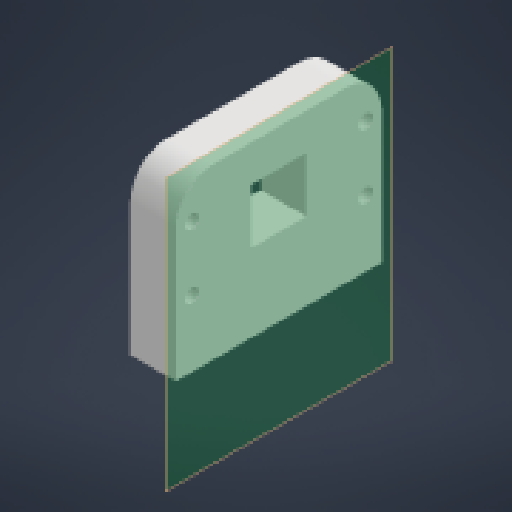
# Autodesk Inventor part: upper_cup
Saved by Autodesk Inventor 2024 (Build 280153000, 153)
## iProperties
Created: 2023-11-08
Part Number: upper_cup
Material: Типовые
Document SubType Name: Modeling
Designer: user
Density: 1 g/cm^3
Appearance: По умолчанию
Author: user
Autodesk Inventor part; units mm, degrees
ref_plane "YZ Plane" through (0, 0, 0) normal (1, 0, 0) x (0, 1, 0)
ref_plane "XZ Plane" through (0, 0, 0) normal (0, 1, 0) x (-1, 0, 0)
ref_plane "XY Plane" through (0, 0, 0) normal (0, 0, 1) x (1, 0, 0)
ref_plane "РабПлоскость1" through (-32.5, 0, 7) normal (-1, 0, 0) x (0, 1, 0)
sketch "Эскиз1" plane through (-32.5, 0, 7) normal (-1, 0, 0) x (0, 1, 0)
  line L0 (15, -5) -> (15, -24) projected
  arc A0 (15, -5) -> (15, 5) centre (15, 0) ccw projected
  line L1 (15, -24) -> (-15, -24) projected
  arc A1 (14.5, -30) -> (22.5, -22) centre (14.5, -22) ccw projected
  line L2 (-14.5, -30) -> (14.5, -30) projected
  arc A2 (-22.5, -22) -> (-14.5, -30) centre (-14.5, -22) ccw projected
  circle A3 centre (-19, -21.5) radius 1.5 projected
  circle A4 centre (-19, -7.5) radius 1.5 projected
  circle A5 centre (19, -21.5) radius 1.5 projected
  circle A6 centre (19, -7.5) radius 1.5 projected
  line L3 (-15, -24) -> (-15, 24) construction
  line L4 (-22.5, 24) -> (-22.5, -22) construction
  line L5 (22.5, -22) -> (22.5, 24) construction
  line L6 (15, 24) -> (15, 5) construction
  line L7 (22.5, -22) -> (22.5, 7)
  line L8 (14, 7) -> (-14, 7) projected
  line L9 (14, 7) -> (22.5, 7)
  line L10 (-14, 7) -> (-15, 7)
  line L11 (-15, 7) -> (-15, -24)
  line L12 (-22.5, -22) -> (-22.5, 7)
  line L13 (-22.5, 7) -> (-15, 7)
  line L14 (15, 5) -> (15, 7)
  line L15 (-6, -22) -> (6, -22)
  line L16 (6, -22) -> (6, -10)
  line L17 (6, -10) -> (-6, -10)
  line L18 (-6, -10) -> (-6, -22)
  point P0 (0, 7)
  point P1 (0, -10)
  dimension "d0" = 2
  dimension "d1" = 12
  dimension "d2" = 12
  constraints: 22 end point, 7 point on line, 3 perpendicular, 2 parallel, 1 collinear, 1 horizontal, 1 midpoint, 1 vertical alignment
  measures "d0" vertical distance of L1.end L15.start
  measures "d1" distance of L16.end L17.end
  measures "d2" distance of L17.end L15.start
extrude "Выдавливание1" add sketch "Эскиз1" along normal blind 10
sketch "Эскиз2" plane through (-32.5, -22.5, 0) normal (0, 0, -1) x (-1, 0, 0)
  arc A0 (7, 34.4641) -> (7, 27.5359) centre (5, 31) ccw projected
  arc A1 (7, 17.4641) -> (7, 10.5359) centre (5, 14) ccw projected
  arc A2 (7, 27.5359) -> (7, 34.4641) centre (5, 31) ccw
  arc A3 (7, 10.5359) -> (7, 17.4641) centre (5, 14) ccw
  point P0 (-32.5, 22.5)
  constraints: 4 point on circle, 2 centre point, 2 concentric
extrude "Выдавливание2" cut sketch "Эскиз2" against normal blind 10
equation "\"d2\" = d1"
